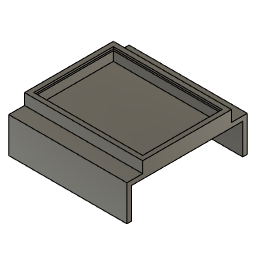
esp_board_holder (Autodesk Fusion 360 design; units mm, degrees)
Autodesk Fusion 360 part; units mm, degrees
sketch "Sketch3" plane through (0, 0, 0) normal (0, 0, 1) x (1, 0, 0)
  line L0 (0, 0) -> (76.5, 0)
  line L1 (76.5, 0) -> (76.5, 3)
  line L2 (76.5, 3) -> (0, 3)
  line L3 (0, 3) -> (0, 0)
  line L4 (0, 75) -> (76.5, 75)
  line L5 (76.5, 75) -> (76.5, 77.9078)
  line L6 (76.5, 77.9078) -> (0, 77.9078)
  line L7 (0, 77.9078) -> (0, 75)
  dimension "d24" = 76.5
  dimension "d25" = 3
  dimension "d26" = 76.5
  dimension "d27" = 72
  constraint horizontal L0
  constraint vertical L1
  constraint horizontal L2
  constraint vertical L3
  constraint coincident L0.start L3.end
  constraint horizontal L4
  constraint vertical L5
  constraint horizontal L6
  constraint vertical L7
  measures "d24" distance of L0.start L0.end
  measures "d25" distance of L0 L2
  measures "d26" distance of L4.start L4.end
  measures "d27" distance of L2 L4
extrude "Extrude4" add sketch "Sketch3" along normal blind 20 makes body 1 at (51, 3, 13.3333) makes body 2 at (51, 77.9078, 13.3333)
sketch "Sketch4" plane through (0, 0, 20) normal (0, 0, 1) x (-1, 0, 0)
  line L0 (0, -3) -> (0, 0)
  line L1 (0, 0) -> (-76.5, 0)
  line L2 (-76.5, 0) -> (-76.5, -3)
  line L3 (-76.5, -3) -> (0, -3)
  line L4 (0, -77.9078) -> (0, -75)
  line L5 (0, -75) -> (-76.5, -75)
  line L6 (-76.5, -75) -> (-76.5, -77.9078)
  line L7 (-76.5, -77.9078) -> (0, -77.9078)
  line L8 (0, -77.9078) -> (-76.5, -77.9078)
  line L9 (-76.5, -77.9078) -> (-76.5, 0)
  line L10 (-76.5, 0) -> (0, 0)
  line L11 (0, 0) -> (0, -77.9078)
  constraint horizontal L8
  constraint vertical L9
  constraint horizontal L10
  constraint vertical L11
  constraint coincident L1.end L2.start
  constraint coincident L4.start L7.end
extrude "Extrude5" add sketch "Sketch4" along normal blind 3 bodies 1 2
sketch "Sketch5" plane through (0, 0, 23) normal (0, 0, 1) x (-1, 0, 0)
  line L0 (0, 0) -> (-76.5, 0)
  line L1 (-76.5, 0) -> (-76.5, -77.9078)
  line L2 (-76.5, -77.9078) -> (0, -77.9078)
  line L3 (0, -77.9078) -> (0, 0)
  line L4 (0, -77.9078) -> (-76.5, 0) construction
  line L5 (-73.5, -64.7039) -> (-3, -64.7039)
  line L6 (-3, -64.7039) -> (-3, -13.2039)
  line L7 (-3, -13.2039) -> (-73.5, -13.2039)
  line L8 (-73.5, -13.2039) -> (-73.5, -64.7039)
  line L9 (-73.5, -64.7039) -> (-3, -13.2039) construction
  line L10 (-3, -64.7039) -> (-73.5, -13.2039) construction
  line L11 (-4, -14.2039) -> (-72.5, -14.2039)
  line L12 (-72.5, -14.2039) -> (-72.5, -63.7039)
  line L13 (-72.5, -63.7039) -> (-4, -63.7039)
  line L14 (-4, -63.7039) -> (-4, -14.2039)
  line L15 (0, -10.2039) -> (-76.5, -10.2039)
  line L16 (-76.5, -10.2039) -> (-76.5, -67.7039)
  line L17 (-76.5, -67.7039) -> (0, -67.7039)
  line L18 (0, -67.7039) -> (0, -10.2039)
  point P0 (-38.25, -38.9539)
  dimension "d35" = 70.5
  dimension "d36" = 51.5
  dimension "d38" = 3
  constraint coincident L2.end L3.start
  constraint coincident L0.end L1.start
  constraint horizontal L5
  constraint perpendicular L5 L6
  constraint parallel L5 L7
  constraint parallel L6 L8
  constraint coincident L9 P0
  constraint coincident L10 P0
  constraint midpoint L4 P0
  measures "d35" distance of L6.end L7.end
  measures "d36" distance of L5.end L6.end
extrude "Extrude8" add sketch "Sketch5" along normal blind 7.25 contours L1 L3 L15 L16 L17 L18 bodies 1
extrude "Extrude9" add sketch "Sketch5" along normal blind 6 contours L5 L6 L7 L8 bodies 1
extrude "Extrude6" [suppressed]
extrude "Extrude7" [suppressed]
equation "board_width = 51 mm"
equation "board_length = 70 mm"
equation "tolerance = 0.25 mm"
equation "board_holder_depth = 6 mm"
equation "board_thickness = 1.25 mm"
equation "board_overhang = 1 mm"
equation "thickness = 3 mm"
equation "bottom_part_gap = 72 mm"
equation "bottom_part_height = 20 mm"
equation "d24 = board_length + thickness * 2 + tolerance * 2"
equation "d25 = thickness"
equation "d26 = board_length + thickness * 2 + tolerance * 2"
equation "d27 = bottom_part_gap"
equation "d28 = bottom_part_height"
equation "d30 = thickness"
equation "d33 = board_holder_depth + board_thickness"
equation "d35 = board_length + tolerance * 2"
equation "d36 = board_width + tolerance * 2"
equation "d37 = -board_overhang"
equation "d38 = thickness"
equation "d39 = board_holder_depth"
equation "d41 = board_holder_depth + board_thickness"
equation "d43 = board_holder_depth"
